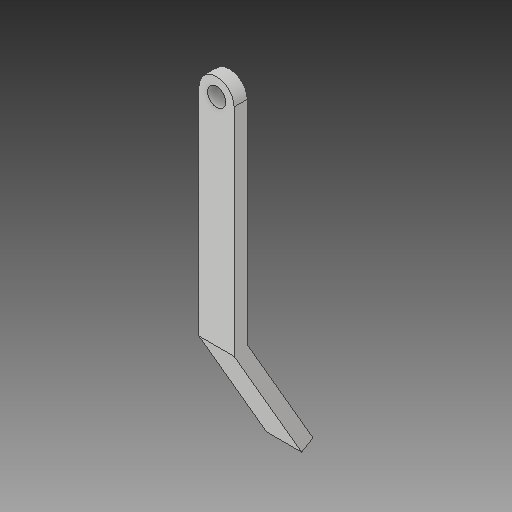
# Autodesk Inventor part: Thumb
Saved by Autodesk Inventor 2017 (Build 210142000, 142)
## iProperties
Created: 2018-11-14
Part Number: Thumb
Material: Generic
Document SubType Name: Modeling
Designer: malik
Density: 1 g/cm^3
Appearance: Default
Author: malik
Autodesk Inventor part; units mm, degrees
ref_plane "YZ Plane" through (0, 0, 0) normal (1, 0, 0) x (0, 1, 0)
ref_plane "XZ Plane" through (0, 0, 0) normal (0, 1, 0) x (-1, 0, 0)
ref_plane "XY Plane" through (0, 0, 0) normal (0, 0, 1) x (1, 0, 0)
sketch "Sketch1" plane through (0, 0, 0) normal (0, 0, 1) x (1, 0, 0)
  circle A0 centre (0, 0) radius 2.0828
  dimension "d0" = 4.1656
  constraints: 1 centre point, 1 coincident
  measures "d0" diameter of A0
sketch "Sketch2" plane through (0, 0, 0) normal (0, 0, 1) x (1, 0, 0)
  circle A0 centre (0, 0) radius 4
  dimension "d1" = 8
  constraints: 1 centre point, 1 coincident
  measures "d1" diameter of A0
extrude "Extrusion1" add sketch "Sketch2" along normal blind 3
sketch "Sketch3" plane through (0, 0, 3) normal (0, 0, 1) x (1, 0, 0)
  circle A0 centre (0, 0) radius 4 projected
  line L0 (-4, 0) -> (4, 0)
  line L1 (4, 0) -> (4, -70)
  line L2 (4, -70) -> (-4, -70)
  line L3 (-4, -70) -> (-4, 0)
  dimension "d4" = 70
  constraints: 8 end point, 2 parallel, 2 point on circle, 1 horizontal, 1 perpendicular
  measures "d4" distance of L0.end L1.end
extrude "Extrusion2" add sketch "Sketch3" against normal blind 3 contours L1 L2 L3 A0
extrude "Extrusion3" cut sketch "Sketch1" along normal blind 5
sketch "Sketch4" plane through (-4, -70, 3) normal (-1, 0, 0) x (0, 0, 1)
  line L0 (-3, 0) -> (-3, 70) projected
  line L1 (-3, 0) -> (-15.5, 0)
  line L2 (-15.5, 0) -> (-3, 21.5912)
  line L3 (-15.5, 0) -> (-12.9037, -1.5031)
  line L4 (-12.9037, -1.5031) -> (-3, 15.6035)
  dimension "d9" = 12.5
  dimension "d10" = 3
  constraints: 8 end point, 2 point on line, 1 horizontal, 1 perpendicular
  measures "d9" distance of L0.start L1.end
  measures "d10" distance of L1.end L3.end
extrude "Extrusion4" add sketch "Sketch4" against normal blind 8 contours L4 L1 L2 L0 | L4 L3 L1
sketch "Sketch5" plane through (-4, -70, 3) normal (-1, 0, 0) x (0, 0, 1)
  line L0 (-3, 15.6035) -> (-12.9037, -1.5031) projected
  line L1 (-3.8073, 14.2091) -> (2.2743, 24.7138)
  line L2 (2.2743, 24.7138) -> (2.8326, -0.03)
  line L3 (2.8326, -0.03) -> (-4.8388, -0.2031)
  line L4 (-4.8388, -0.2031) -> (-3.8073, 14.2091)
  point P0 (-3, 70)
  constraints: 8 end point, 1 collinear, 1 point on line
extrude "Extrusion5" cut sketch "Sketch5" against normal blind 8
sketch "Sketch6" plane through (-4, -70, -12.5) normal (0, -0.8654, -0.501) x (1, 0, 0)
  line L0 (0, 0) -> (0, 3) projected
  line L1 (8, 0) -> (0, 0) projected
  line L2 (0, 0) -> (8, 0)
  line L3 (8, 0) -> (8, 3)
  line L4 (8, 3) -> (0, 3)
  line L5 (0, 3) -> (0, 0)
  point P0 (4, -24.2544)
  constraints: 8 end point, 3 equal length, 1 perpendicular
extrude "Extrusion6" add sketch "Sketch6" along normal blind 5
body "Solid1"
